Autodesk Fusion 360 part; units mm, degrees
(part 4 of 8)
  line L112 (-117.1979, 4.132) -> (-121.8798, -2.8001)
  spline S456 degree 3 poles (-131.6156, -11.2139) (-132.3559, -11.2139) (-133.0961, -11.2403) (-133.4953, -11.2934) knots 0 0 0 0 1 1 1 1
  spline S457 degree 3 poles (-133.4953, -11.2934) (-133.0961, -11.2403) (-132.3559, -11.2139) (-131.6156, -11.2139) knots -1 -1 -1 -1 0 0 0 0
  spline S458 degree 3 poles (188.5245, 6.5131) (188.7626, 6.5131) (189.0272, 5.9575) (189.0272, 5.64) knots 0 0 0 0 1 1 1 1
  spline S459 degree 3 poles (189.0272, 5.64) (189.0272, 5.9575) (188.7626, 6.5131) (188.5245, 6.5131) knots -1 -1 -1 -1 0 0 0 0
  spline S460 degree 3 poles (159.7907, 5.6135) (159.7907, 5.9575) (160.0818, 6.5131) (160.2934, 6.5131) knots 0 0 0 0 1 1 1 1
  spline S461 degree 3 poles (160.2934, 6.5131) (160.0818, 6.5131) (159.7907, 5.9575) (159.7907, 5.6135) knots -1 -1 -1 -1 0 0 0 0
  spline S462 degree 3 poles (213.7393, -9.3619) (215.3268, -9.3619) (215.6707, -9.4148) (215.6707, -8.7798) knots 0 0 0 0 1 1 1 1
  line L113 (215.6707, -8.7798) -> (215.6707, -3.1442)
  line L114 (215.6707, -3.1442) -> (213.8186, -3.1971)
  spline S463 degree 3 poles (213.8186, -3.1971) (211.6491, -3.25) (211.8078, -5.9753) (211.0141, -5.9753) knots 0 0 0 0 1 1 1 1
  spline S464 degree 3 poles (211.0141, -5.9753) (210.6966, -5.9753) (210.1145, -5.6842) (210.1145, -5.4725) knots 0 0 0 0 1 1 1 1
  spline S465 degree 3 poles (210.1145, -5.4725) (210.2468, -3.303) (210.2468, -1.1334) (210.1145, 1.0362) knots 0 0 0 0 1 1 1 1
  spline S466 degree 3 poles (210.1145, 1.0362) (210.1145, 1.2479) (210.6966, 1.5389) (211.0141, 1.5389) knots 0 0 0 0 1 1 1 1
  spline S467 degree 3 poles (211.0141, 1.5389) (211.8078, 1.5389) (211.6491, -1.1863) (213.8186, -1.2392) knots 0 0 0 0 1 1 1 1
  line L115 (213.8186, -1.2392) -> (215.6707, -1.2921)
  line L116 (215.6707, -1.2921) -> (215.6707, 4.1583)
  spline S468 degree 3 poles (215.6707, 4.1583) (215.6707, 5.296) (214.2155, 5.2166) (214.2155, 5.6135) knots 0 0 0 0 1 1 1 1
  spline S469 degree 3 poles (214.2155, 5.6135) (214.2155, 5.9575) (214.5066, 6.5131) (214.7182, 6.5131) knots 0 0 0 0 1 1 1 1
  spline S470 degree 3 poles (214.7182, 6.5131) (215.7501, 6.4602) (217.0466, 6.4337) (218.3166, 6.4337) knots 0 0 0 0 1 1 1 1
  spline S471 degree 3 poles (218.3166, 6.4337) (219.613, 6.4337) (220.883, 6.4602) (221.9414, 6.5131) knots 0 0 0 0 1 1 1 1
  spline S472 degree 3 poles (221.9414, 6.5131) (222.1795, 6.5131) (222.4441, 5.9575) (222.4441, 5.64) knots 0 0 0 0 1 1 1 1
  spline S473 degree 3 poles (222.4441, 5.64) (222.4441, 5.2166) (221.0153, 5.296) (221.0153, 4.1583) knots 0 0 0 0 1 1 1 1
  line L117 (221.0153, 4.1583) -> (221.0153, -8.9386)
  spline S474 degree 3 poles (221.0153, -8.9386) (221.0153, -10.0763) (222.4441, -9.9969) (222.4441, -10.3938) knots 0 0 0 0 1 1 1 1
  spline S475 degree 3 poles (222.4441, -10.3938) (222.4441, -10.7113) (222.1795, -11.2934) (221.9414, -11.2934) knots 0 0 0 0 1 1 1 1
  spline S476 degree 3 poles (221.9414, -11.2934) (220.1951, -11.2405) (217.7874, -11.214) (215.3532, -11.214) knots 0 0 0 0 1 1 1 1
  spline S477 degree 3 poles (215.3532, -11.214) (212.628, -11.214) (209.8764, -11.2405) (207.9184, -11.2934) knots 0 0 0 0 1 1 1 1
  spline S478 degree 3 poles (207.9184, -11.2934) (207.3893, -11.3225) (207.0718, -11.1611) (207.0718, -10.6848) knots 0 0 0 0 1 1 1 1
  spline S479 degree 3 poles (207.0718, -10.6848) (207.0718, -10.1028) (207.4951, -6.9807) (207.4951, -6.769) knots 0 0 0 0 1 1 1 1
  spline S480 degree 3 poles (207.4951, -6.769) (207.4951, -6.5573) (208.0507, -6.2663) (208.3682, -6.2663) knots 0 0 0 0 1 1 1 1
  spline S481 degree 3 poles (208.3682, -6.2663) (208.8709, -6.2663) (208.9503, -9.3619) (213.7393, -9.3619) knots 0 0 0 0 1 1 1 1
  spline S482 degree 3 poles (110.3163, 6.4337) (111.0571, 6.4337) (111.798, 6.4602) (112.1948, 6.5131) knots 0 0 0 0 1 1 1 1
  spline S483 degree 3 poles (112.1948, 6.5131) (111.798, 6.4602) (111.0571, 6.4337) (110.3163, 6.4337) knots -1 -1 -1 -1 0 0 0 0
  spline S484 degree 3 poles (106.0036, -11.2934) (105.104, -11.2934) (104.8394, -11.1346) (104.6542, -10.6584) knots 0 0 0 0 1 1 1 1
  spline S485 degree 3 poles (104.6542, -10.6584) (104.8394, -11.1346) (105.104, -11.2934) (106.0036, -11.2934) knots -1 -1 -1 -1 0 0 0 0
  spline S486 degree 3 poles (213.7393, -9.3619) (215.3268, -9.3619) (215.6707, -9.4148) (215.6707, -8.7798) knots 0 0 0 0 1 1 1 1
  spline S487 degree 3 poles (215.6707, -8.7798) (215.6707, -9.4148) (215.3268, -9.3619) (213.7393, -9.3619) knots -1 -1 -1 -1 0 0 0 0
  spline S488 degree 3 poles (177.3326, 5.64) (177.3326, 5.2166) (175.9039, 5.296) (175.9039, 4.1583) knots 0 0 0 0 1 1 1 1
  spline S489 degree 3 poles (175.9039, 4.1583) (175.9039, 5.296) (177.3326, 5.2166) (177.3326, 5.64) knots -1 -1 -1 -1 0 0 0 0
  spline S490 degree 3 poles (181.3014, -11.2934) (181.0897, -11.3225) (180.7986, -10.7378) (180.7986, -10.4203) knots 0 0 0 0 1 1 1 1
  spline S491 degree 3 poles (180.7986, -10.4203) (180.7986, -10.7378) (181.0897, -11.3225) (181.3014, -11.2934) knots -1 -1 -1 -1 0 0 0 0
  spline S492 degree 3 poles (-119.8955, 6.5132) (-119.4963, 6.4601) (-118.756, 6.4338) (-118.0157, 6.4338) knots 0 0 0 0 1 1 1 1
  spline S493 degree 3 poles (-118.0157, 6.4338) (-118.756, 6.4338) (-119.4963, 6.4601) (-119.8955, 6.5132) knots -1 -1 -1 -1 0 0 0 0
  line L118 (-132.8326, 4.1584) -> (-128.3096, -2.7738)
  line L119 (-128.3096, -2.7738) -> (-132.8326, 4.1584)
  spline S494 degree 3 poles (95.6584, -10.6584) (95.4732, -11.1346) (95.235, -11.2934) (94.309, -11.2934) knots 0 0 0 0 1 1 1 1
  spline S495 degree 3 poles (94.309, -11.2934) (95.235, -11.2934) (95.4732, -11.1346) (95.6584, -10.6584) knots -1 -1 -1 -1 0 0 0 0
  spline S496 degree 3 poles (163.9182, 6.4337) (165.2147, 6.4337) (166.4873, 6.4602) (167.5457, 6.5131) knots 0 0 0 0 1 1 1 1
  spline S497 degree 3 poles (167.5457, 6.5131) (166.4873, 6.4602) (165.2147, 6.4337) (163.9182, 6.4337) knots -1 -1 -1 -1 0 0 0 0
  spline S498 degree 3 poles (211.0141, -5.9753) (210.6966, -5.9753) (210.1145, -5.6842) (210.1145, -5.4725) knots 0 0 0 0 1 1 1 1
  spline S499 degree 3 poles (210.1145, -5.4725) (210.1145, -5.6842) (210.6966, -5.9753) (211.0141, -5.9753) knots -1 -1 -1 -1 0 0 0 0
  spline S500 degree 3 poles (102.0084, 6.4337) (102.6698, 6.4337) (103.3313, 6.4602) (104.2573, 6.5131) knots 0 0 0 0 1 1 1 1
  spline S501 degree 3 poles (104.2573, 6.5131) (103.3313, 6.4602) (102.6698, 6.4337) (102.0084, 6.4337) knots -1 -1 -1 -1 0 0 0 0
  spline S502 degree 3 poles (-4.0362, 6.4867) (-2.3431, 6.4867) (-3.3764, 5.8779) (-2.1844, 4.1319) knots 0 0 0 0 1 1 1 1
  spline S503 degree 3 poles (-2.1844, 4.1319) (-3.3764, 5.8779) (-2.3431, 6.4867) (-4.0362, 6.4867) knots -1 -1 -1 -1 0 0 0 0
  spline S504 degree 3 poles (221.9414, -11.2934) (220.1951, -11.2405) (217.7874, -11.214) (215.3532, -11.214) knots 0 0 0 0 1 1 1 1
  spline S505 degree 3 poles (215.3532, -11.214) (217.7874, -11.214) (220.1951, -11.2405) (221.9414, -11.2934) knots -1 -1 -1 -1 0 0 0 0
  spline S506 degree 3 poles (168.0193, 5.64) (168.0193, 5.2166) (166.5905, 5.296) (166.5905, 4.1583) knots 0 0 0 0 1 1 1 1
  spline S507 degree 3 poles (166.5905, 4.1583) (166.5905, 5.296) (168.0193, 5.2166) (168.0193, 5.64) knots -1 -1 -1 -1 0 0 0 0
  spline S508 degree 3 poles (94.309, -11.2934) (93.4094, -11.2934) (91.6367, -11.1346) (89.7317, -11.2934) knots 0 0 0 0 1 1 1 1
  spline S509 degree 3 poles (89.7317, -11.2934) (91.6367, -11.1346) (93.4094, -11.2934) (94.309, -11.2934) knots -1 -1 -1 -1 0 0 0 0
  spline S510 degree 3 poles (160.2934, 6.5131) (161.3253, 6.4602) (162.6218, 6.4337) (163.9182, 6.4337) knots 0 0 0 0 1 1 1 1
  spline S511 degree 3 poles (163.9182, 6.4337) (162.6218, 6.4337) (161.3253, 6.4602) (160.2934, 6.5131) knots -1 -1 -1 -1 0 0 0 0
  spline S512 degree 3 poles (167.5457, -11.2934) (166.4873, -11.2405) (165.2147, -11.214) (163.9182, -11.214) knots 0 0 0 0 1 1 1 1
  spline S513 degree 3 poles (163.9182, -11.214) (165.2147, -11.214) (166.4873, -11.2405) (167.5457, -11.2934) knots -1 -1 -1 -1 0 0 0 0
  spline S514 degree 3 poles (-63.4057, -10.3935) (-63.4057, -10.5655) (-63.4913, -10.8075) (-63.6031, -10.9931) knots 0 0 0 0 0.541892 0.541892 0.541892 0.541892
  spline S515 degree 3 poles (-63.6031, -10.9931) (-63.4913, -10.8075) (-63.4057, -10.5655) (-63.4057, -10.3935) knots -0.541892 -0.541892 -0.541892 -0.541892 0 0 0 0
  spline S516 degree 3 poles (-79.7806, -11.1902) (-80.577, -11.1902) (-81.3698, -11.2136) (-81.768, -11.2666) knots 0 0 0 0 1 1 1 1
  spline S517 degree 3 poles (-81.768, -11.2666) (-81.3698, -11.2136) (-80.577, -11.1902) (-79.7806, -11.1902) knots -1 -1 -1 -1 0 0 0 0
  spline S518 degree 5 poles (-63.6031, -10.9931) (-63.6143, -11.005) (-63.6642, -11.057) (-63.7203, -11.1105) (-63.7825, -11.1656) (-63.8508, -11.2222) (-63.907, -11.2666) knots 0.913312 0.913312 0.913312 0.913312 0.913312 0.913312 0.933333 1 1 1 1 1 1
  spline S519 degree 5 poles (-63.907, -11.2666) (-63.8508, -11.2222) (-63.7825, -11.1656) (-63.7203, -11.1105) (-63.6642, -11.057) (-63.6143, -11.005) (-63.6031, -10.9931) knots -1 -1 -1 -1 -1 -1 -0.933333 -0.913312 -0.913312 -0.913312 -0.913312 -0.913312 -0.913312
  spline S520 degree 3 poles (-44.0427, -6.2399) (-44.0427, -6.0282) (-43.4578, -5.7371) (-43.1421, -5.7371) knots 0 0 0 0 1 1 1 1
  spline S521 degree 3 poles (-43.1421, -5.7371) (-43.4578, -5.7371) (-44.0427, -6.0282) (-44.0427, -6.2399) knots -1 -1 -1 -1 0 0 0 0
  spline S522 degree 3 poles (23.2168, -2.3771) (23.2168, -7.2718) (22.1298, -9.7058) (19.7498, -9.7058) knots -1 -1 -1 -1 0 0 0 0
  spline S523 degree 3 poles (23.2168, -2.3771) (23.2168, -7.2718) (22.1298, -9.7058) (19.7498, -9.7058) knots -1 -1 -1 -1 0 0 0 0
  line L120 (-37.7953, 4.1582) -> (-37.7953, -8.7797)
  line L121 (-37.7953, -8.7797) -> (-37.7953, 4.1582)
  spline S524 degree 3 poles (19.7498, 4.9254) (22.1298, 4.9254) (23.2168, 2.518) (23.2168, -2.3771) knots -1 -1 -1 -1 0 0 0 0
  spline S525 degree 3 poles (19.7498, 4.9254) (22.1298, 4.9254) (23.2168, 2.518) (23.2168, -2.3771) knots -1 -1 -1 -1 0 0 0 0
  spline S526 degree 3 poles (-38.6427, -9.3619) (-38.111, -9.3619) (-37.7953, -9.4413) (-37.7953, -8.7797) knots 0 0 0 0 1 1 1 1
  line L122 (-37.7953, -8.7797) -> (-37.7953, 4.1582)
  spline S527 degree 3 poles (-37.7953, 4.1582) (-37.7953, 5.296) (-39.2508, 5.2166) (-39.2508, 5.6137) knots 0 0 0 0 1 1 1 1
  spline S528 degree 3 poles (-39.2508, 5.6137) (-39.2508, 5.931) (-38.9584, 6.5132) (-38.7457, 6.5132) knots 0 0 0 0 1 1 1 1
  spline S529 degree 3 poles (-38.7457, 6.5132) (-37.7156, 6.46) (-36.4196, 6.4338) (-35.1236, 6.4338) knots 0 0 0 0 1 1 1 1
  spline S530 degree 3 poles (-35.1236, 6.4338) (-33.8243, 6.4338) (-32.5549, 6.46) (-31.4982, 6.5132) knots 0 0 0 0 1 1 1 1
  spline S531 degree 3 poles (-31.4982, 6.5132) (-31.2855, 6.5132) (-31.0197, 5.931) (-31.0197, 5.6137) knots 0 0 0 0 1 1 1 1
  spline S532 degree 3 poles (-31.0197, 5.6137) (-31.0197, 5.2166) (-32.4486, 5.296) (-32.4486, 4.1582) knots 0 0 0 0 1 1 1 1
  line L123 (-32.4486, 4.1582) -> (-32.4486, -8.7797)
  spline S533 degree 3 poles (-32.4486, -8.7797) (-32.4486, -9.1768) (-32.1329, -9.3619) (-31.4184, -9.3619) knots 0 0 0 0 1 1 1 1
  spline S534 degree 3 poles (-31.4184, -9.3619) (-28.3745, -9.3619) (-27.1051, -5.7372) (-26.6033, -5.7372) knots 0 0 0 0 1 1 1 1
  spline S535 degree 3 poles (-26.6033, -5.7372) (-26.2843, -5.7372) (-25.7028, -6.0017) (-25.7028, -6.2399) knots 0 0 0 0 1 1 1 1
  spline S536 degree 3 poles (-25.7028, -6.2399) (-25.7028, -6.4516) (-26.2046, -10.1292) (-26.2578, -10.4731) knots 0 0 0 0 1 1 1 1
  spline S537 degree 3 poles (-26.2578, -10.4731) (-26.3641, -11.161) (-26.63, -11.3225) (-27.1849, -11.2933) knots 0 0 0 0 1 1 1 1
  spline S538 degree 3 poles (-27.1849, -11.2933) (-29.9364, -11.2404) (-32.6613, -11.2138) (-35.3861, -11.2138) knots 0 0 0 0 1 1 1 1
  spline S539 degree 3 poles (-35.3861, -11.2138) (-38.111, -11.2138) (-40.8658, -11.2404) (-43.5907, -11.2933) knots 0 0 0 0 1 1 1 1
  spline S540 degree 3 poles (-43.5907, -11.2933) (-44.1191, -11.3225) (-44.4381, -11.161) (-44.4381, -10.6848) knots 0 0 0 0 1 1 1 1
  spline S541 degree 3 poles (-44.4381, -10.6848) (-44.4381, -10.1292) (-44.0427, -6.4516) (-44.0427, -6.2399) knots 0 0 0 0 1 1 1 1
  spline S542 degree 3 poles (-44.0427, -6.2399) (-44.0427, -6.0282) (-43.4578, -5.7371) (-43.1421, -5.7371) knots 0 0 0 0 1 1 1 1
  spline S543 degree 3 poles (-43.1421, -5.7371) (-42.6404, -5.7371) (-42.4277, -9.3619) (-38.6427, -9.3619) knots 0 0 0 0 1 1 1 1
  spline S544 degree 3 poles (177.3326, -10.4203) (177.3326, -10.7378) (177.068, -11.3225) (176.8564, -11.2934) knots 0 0 0 0 1 1 1 1
  spline S545 degree 3 poles (176.8564, -11.2934) (177.068, -11.3225) (177.3326, -10.7378) (177.3326, -10.4203) knots -1 -1 -1 -1 0 0 0 0
  spline S546 degree 3 poles (11.3616, 8.4444) (11.3616, 10.4553) (12.9234, 12.1751) (15.2526, 12.1222) knots 0 0 0 0 1 1 1 1
  spline S547 degree 3 poles (15.2526, 12.1222) (12.9234, 12.1751) (11.3616, 10.4553) (11.3616, 8.4444) knots -1 -1 -1 -1 0 0 0 0
  spline S548 degree 3 poles (-25.7028, -6.2399) (-25.7028, -6.4516) (-26.2046, -10.1292) (-26.2578, -10.4731) knots 0 0 0 0 1 1 1 1
  spline S549 degree 3 poles (-26.2578, -10.4731) (-26.2046, -10.1292) (-25.7028, -6.4516) (-25.7028, -6.2399) knots -1 -1 -1 -1 0 0 0 0
  spline S550 degree 3 poles (24.1426, 7.307) (24.8832, 7.307) (25.2803, 7.8624) (25.2803, 8.4181) knots 0 0 0 0 1 1 1 1
  spline S551 degree 3 poles (25.2803, 8.4181) (25.2803, 7.8624) (24.8832, 7.307) (24.1426, 7.307) knots -1 -1 -1 -1 0 0 0 0
  spline S552 degree 3 poles (19.5885, -11.5568) (19.4017, -11.5543) (19.2169, -11.5473) (19.0342, -11.5361) knots 0.009853 0.009853 0.009853 0.009853 0.044162 0.044162 0.044162 0.044162
  spline S553 degree 3 poles (19.0342, -11.5361) (19.2169, -11.5473) (19.4017, -11.5543) (19.5885, -11.5568) knots -0.044162 -0.044162 -0.044162 -0.044162 -0.009853 -0.009853 -0.009853 -0.009853
  spline S554 degree 3 poles (-31.0197, 5.6137) (-31.0197, 5.2166) (-32.4486, 5.296) (-32.4486, 4.1582) knots 0 0 0 0 1 1 1 1
  spline S555 degree 3 poles (-32.4486, 4.1582) (-32.4486, 5.296) (-31.0197, 5.2166) (-31.0197, 5.6137) knots -1 -1 -1 -1 0 0 0 0
  spline S556 degree 3 poles (215.6707, 4.1583) (215.6707, 5.296) (214.2155, 5.2166) (214.2155, 5.6135) knots 0 0 0 0 1 1 1 1
  spline S557 degree 3 poles (214.2155, 5.6135) (214.2155, 5.2166) (215.6707, 5.296) (215.6707, 4.1583) knots -1 -1 -1 -1 0 0 0 0
  spline S558 degree 3 poles (-21.7884, -11.0288) (-22.4483, -11.0288) (-22.6342, -11.2934) (-23.0859, -11.2934) knots 0 0 0 0 1 1 1 1
  spline S559 degree 3 poles (-23.0859, -11.2934) (-22.6342, -11.2934) (-22.4483, -11.0288) (-21.7884, -11.0288) knots -1 -1 -1 -1 0 0 0 0
  spline S560 degree 3 poles (299.0115, 4.1318) (298.6411, 5.2166) (297.4505, 5.1902) (297.4505, 5.587) knots 0 0 0 0 1 1 1 1
  spline S561 degree 3 poles (297.4505, 5.587) (297.4505, 5.1902) (298.6411, 5.2166) (299.0115, 4.1318) knots -1 -1 -1 -1 0 0 0 0
  line L124 (-128.3096, -2.7738) -> (-132.4373, -8.9121)
  line L125 (-132.4373, -8.9121) -> (-128.3096, -2.7738)
  line L126 (-52.1084, -0.3134) -> (-52.1084, -8.9652)
  line L127 (-52.1084, -8.9652) -> (-52.1084, -0.3134)
  spline S562 degree 3 poles (-53.0631, -11.2935) (-53.2726, -11.2935) (-53.5645, -10.7379) (-53.5645, -10.4202) knots 0 0 0 0 1 1 1 1
  spline S563 degree 3 poles (-53.5645, -10.4202) (-53.5645, -10.7379) (-53.2726, -11.2935) (-53.0631, -11.2935) knots -1 -1 -1 -1 0 0 0 0
  line L128 (161.2459, 4.1583) -> (161.2459, -8.965)
  line L129 (161.2459, -8.965) -> (161.2459, 4.1583)
  line L130 (-78.5932, -8.9383) -> (-74.6506, 2.4388)
  line L131 (-74.6506, 2.4388) -> (-78.5932, -8.9383)
  line L132 (8.0583, -8.9652) -> (8.0583, 4.1848)
  line L133 (8.0583, 4.1848) -> (8.0583, -8.9652)
  spline S564 degree 3 poles (184.8997, -11.214) (183.6297, -11.214) (182.3332, -11.2405) (181.3014, -11.2934) knots 0 0 0 0 1 1 1 1
  spline S565 degree 3 poles (181.3014, -11.2934) (182.3332, -11.2405) (183.6297, -11.214) (184.8997, -11.214) knots -1 -1 -1 -1 0 0 0 0
  line L134 (187.5984, -8.965) -> (187.5984, 4.1583)
  line L135 (187.5984, 4.1583) -> (187.5984, -8.965)
  spline S566 degree 3 poles (221.9414, 6.5131) (222.1795, 6.5131) (222.4441, 5.9575) (222.4441, 5.64) knots 0 0 0 0 1 1 1 1
  spline S567 degree 3 poles (222.4441, 5.64) (222.4441, 5.9575) (222.1795, 6.5131) (221.9414, 6.5131) knots -1 -1 -1 -1 0 0 0 0
  spline S568 degree 3 poles (182.2539, 4.1583) (182.2539, 5.296) (180.7986, 5.2166) (180.7986, 5.64) knots 0 0 0 0 1 1 1 1
  spline S569 degree 3 poles (180.7986, 5.64) (180.7986, 5.2166) (182.2539, 5.296) (182.2539, 4.1583) knots -1 -1 -1 -1 0 0 0 0
  line L136 (109.3902, 4.1583) -> (108.2261, -4.7317)
  line L137 (108.2261, -4.7317) -> (109.3902, 4.1583)
  line L138 (213.8186, -3.1971) -> (215.6707, -3.1442)
  line L139 (215.6707, -3.1442) -> (213.8186, -3.1971)
  line L140 (0.9622, -0.5248) -> (-2.1844, 4.1319)
  line L141 (-2.1844, 4.1319) -> (0.9622, -0.5248)
  spline S570 degree 3 poles (207.9184, -11.2934) (207.3893, -11.3225) (207.0718, -11.1611) (207.0718, -10.6848) knots 0 0 0 0 1 1 1 1
  spline S571 degree 3 poles (207.0718, -10.6848) (207.0718, -11.1611) (207.3893, -11.3225) (207.9184, -11.2934) knots -1 -1 -1 -1 0 0 0 0
  line L142 (95.6584, -10.6584) -> (100.1563, 1.6977)
  line L143 (100.1563, 1.6977) -> (95.6584, -10.6584)
  line L144 (166.5905, -8.965) -> (166.5905, 4.1583)
  line L145 (166.5905, 4.1583) -> (166.5905, -8.965)
  spline S572 degree 3 poles (213.8186, -3.1971) (211.6491, -3.25) (211.8078, -5.9753) (211.0141, -5.9753) knots 0 0 0 0 1 1 1 1
  spline S573 degree 3 poles (211.0141, -5.9753) (211.8078, -5.9753) (211.6491, -3.25) (213.8186, -3.1971) knots -1 -1 -1 -1 0 0 0 0
  spline S574 degree 3 poles (9.0107, 6.5131) (9.2223, 6.5131) (9.5118, 5.9573) (9.5118, 5.6398) knots 0 0 0 0 1 1 1 1
  spline S575 degree 3 poles (9.5118, 5.6398) (9.5118, 5.9573) (9.2223, 6.5131) (9.0107, 6.5131) knots -1 -1 -1 -1 0 0 0 0
  spline S576 degree 3 poles (-129.7359, -11.2934) (-130.1351, -11.2403) (-130.8754, -11.2139) (-131.6156, -11.2139) knots 0 0 0 0 1 1 1 1
  spline S577 degree 3 poles (-131.6156, -11.2139) (-130.8754, -11.2139) (-130.1351, -11.2403) (-129.7359, -11.2934) knots -1 -1 -1 -1 0 0 0 0
  spline S578 degree 3 poles (173.2316, 6.4337) (174.5016, 6.4337) (175.798, 6.4602) (176.8564, 6.5131) knots 0 0 0 0 1 1 1 1
  spline S579 degree 3 poles (176.8564, 6.5131) (175.798, 6.4602) (174.5016, 6.4337) (173.2316, 6.4337) knots -1 -1 -1 -1 0 0 0 0
  spline S580 degree 3 poles (-37.7953, -8.7797) (-37.7953, -9.4413) (-38.111, -9.3619) (-38.6427, -9.3619) knots -1 -1 -1 -1 0 0 0 0
  spline S581 degree 3 poles (-38.6427, -9.3619) (-42.4277, -9.3619) (-42.6404, -5.7371) (-43.1421, -5.7371) knots -1 -1 -1 -1 0 0 0 0
  spline S582 degree 3 poles (-43.1421, -5.7371) (-43.4578, -5.7371) (-44.0427, -6.0282) (-44.0427, -6.2399) knots -1 -1 -1 -1 0 0 0 0
  spline S583 degree 3 poles (-44.0427, -6.2399) (-44.0427, -6.4516) (-44.4381, -10.1292) (-44.4381, -10.6848) knots -1 -1 -1 -1 0 0 0 0
  spline S584 degree 3 poles (-44.4381, -10.6848) (-44.4381, -11.161) (-44.1191, -11.3225) (-43.5907, -11.2933) knots -1 -1 -1 -1 0 0 0 0
  spline S585 degree 3 poles (-43.5907, -11.2933) (-40.8658, -11.2404) (-38.111, -11.2138) (-35.3861, -11.2138) knots -1 -1 -1 -1 0 0 0 0
  spline S586 degree 3 poles (-35.3861, -11.2138) (-32.6613, -11.2138) (-29.9364, -11.2404) (-27.1849, -11.2933) knots -1 -1 -1 -1 0 0 0 0
  spline S587 degree 3 poles (-27.1849, -11.2933) (-26.63, -11.3225) (-26.3641, -11.161) (-26.2578, -10.4731) knots -1 -1 -1 -1 0 0 0 0
  spline S588 degree 3 poles (-26.2578, -10.4731) (-26.2046, -10.1292) (-25.7028, -6.4516) (-25.7028, -6.2399) knots -1 -1 -1 -1 0 0 0 0
  spline S589 degree 3 poles (-25.7028, -6.2399) (-25.7028, -6.0017) (-26.2843, -5.7372) (-26.6033, -5.7372) knots -1 -1 -1 -1 0 0 0 0
  spline S590 degree 3 poles (-26.6033, -5.7372) (-27.1051, -5.7372) (-28.3745, -9.3619) (-31.4184, -9.3619) knots -1 -1 -1 -1 0 0 0 0
  spline S591 degree 3 poles (-31.4184, -9.3619) (-32.1329, -9.3619) (-32.4486, -9.1768) (-32.4486, -8.7797) knots -1 -1 -1 -1 0 0 0 0
  line L146 (-32.4486, -8.7797) -> (-32.4486, 4.1582)
  spline S592 degree 3 poles (-32.4486, 4.1582) (-32.4486, 5.296) (-31.0197, 5.2166) (-31.0197, 5.6137) knots -1 -1 -1 -1 0 0 0 0
  spline S593 degree 3 poles (-31.0197, 5.6137) (-31.0197, 5.931) (-31.2855, 6.5132) (-31.4982, 6.5132) knots -1 -1 -1 -1 0 0 0 0
  spline S594 degree 3 poles (-31.4982, 6.5132) (-32.5549, 6.46) (-33.8243, 6.4338) (-35.1236, 6.4338) knots -1 -1 -1 -1 0 0 0 0
  spline S595 degree 3 poles (-35.1236, 6.4338) (-36.4196, 6.4338) (-37.7156, 6.46) (-38.7457, 6.5132) knots -1 -1 -1 -1 0 0 0 0
  spline S596 degree 3 poles (-38.7457, 6.5132) (-38.9584, 6.5132) (-39.2508, 5.931) (-39.2508, 5.6137) knots -1 -1 -1 -1 0 0 0 0
  spline S597 degree 3 poles (-39.2508, 5.6137) (-39.2508, 5.2166) (-37.7953, 5.296) (-37.7953, 4.1582) knots -1 -1 -1 -1 0 0 0 0
  line L147 (-37.7953, 4.1582) -> (-37.7953, -8.7797)
  spline S598 degree 3 poles (12.3354, 3.4367) (13.6571, 5.1309) (15.615, 6.2706) (18.0029, 6.6455) knots 0.475314 0.475314 0.475314 0.475314 1 1 1 1
  spline S599 degree 3 poles (18.0029, 6.6455) (15.615, 6.2706) (13.6571, 5.1309) (12.3354, 3.4367) knots -1 -1 -1 -1 -0.475314 -0.475314 -0.475314 -0.475314
  spline S600 degree 3 poles (24.3785, 5.7192) (25.0522, 5.3732) (25.6655, 4.9493) (26.2098, 4.4555) knots 0 0 0 0 0.233548 0.233548 0.233548 0.233548
  spline S601 degree 3 poles (26.2098, 4.4555) (25.6655, 4.9493) (25.0522, 5.3732) (24.3785, 5.7192) knots -0.233548 -0.233548 -0.233548 -0.233548 0 0 0 0
  spline S602 degree 3 poles (-38.6427, -9.3619) (-38.111, -9.3619) (-37.7953, -9.4413) (-37.7953, -8.7797) knots 0 0 0 0 1 1 1 1
  spline S603 degree 3 poles (-37.7953, -8.7797) (-37.7953, -9.4413) (-38.111, -9.3619) (-38.6427, -9.3619) knots -1 -1 -1 -1 0 0 0 0
  line L148 (-64.9913, -8.9383) -> (-70.4164, 6.5133)
  line L149 (-70.4164, 6.5133) -> (-64.9913, -8.9383)
  spline S604 degree 3 poles (-52.1084, -0.3134) (-52.1084, 2.7559) (-53.434, 4.3435) (-55.6798, 4.3435) knots 0 0 0 0 1 1 1 1
  spline S605 degree 3 poles (-55.6798, 4.3435) (-53.434, 4.3435) (-52.1084, 2.7559) (-52.1084, -0.3134) knots -1 -1 -1 -1 0 0 0 0
  spline S606 degree 3 poles (176.8564, 6.5131) (177.068, 6.5131) (177.3326, 5.9575) (177.3326, 5.64) knots 0 0 0 0 1 1 1 1
  spline S607 degree 3 poles (177.3326, 5.64) (177.3326, 5.9575) (177.068, 6.5131) (176.8564, 6.5131) knots -1 -1 -1 -1 0 0 0 0
  spline S608 degree 3 poles (-32.4486, -8.7797) (-32.4486, -9.1768) (-32.1329, -9.3619) (-31.4184, -9.3619) knots 0 0 0 0 1 1 1 1
  spline S609 degree 3 poles (-31.4184, -9.3619) (-32.1329, -9.3619) (-32.4486, -9.1768) (-32.4486, -8.7797) knots -1 -1 -1 -1 0 0 0 0
  spline S610 degree 3 poles (170.5593, 4.1583) (170.5593, 5.296) (169.1041, 5.2166) (169.1041, 5.64) knots 0 0 0 0 1 1 1 1
  spline S611 degree 3 poles (169.1041, 5.64) (169.1041, 5.2166) (170.5593, 5.296) (170.5593, 4.1583) knots -1 -1 -1 -1 0 0 0 0
  spline S612 degree 3 poles (-133.9953, -10.4202) (-133.9953, -9.9969) (-133.0729, -9.8648) (-132.4373, -8.9121) knots 0 0 0 0 1 1 1 1
  spline S613 degree 3 poles (-132.4373, -8.9121) (-133.0729, -9.8648) (-133.9953, -9.9969) (-133.9953, -10.4202) knots -1 -1 -1 -1 0 0 0 0
  line L150 (182.2539, 4.1583) -> (182.2539, -1.9007)
  line L151 (182.2539, -1.9007) -> (182.2539, 4.1583)
  spline S614 degree 3 poles (169.1041, 5.64) (169.1041, 5.9575) (169.3951, 6.5131) (169.6068, 6.5131) knots 0 0 0 0 1 1 1 1
  spline S615 degree 3 poles (169.6068, 6.5131) (169.3951, 6.5131) (169.1041, 5.9575) (169.1041, 5.64) knots -1 -1 -1 -1 0 0 0 0
  line L152 (182.2539, -1.9007) -> (175.9039, -1.9007)
  line L153 (175.9039, -1.9007) -> (182.2539, -1.9007)
  spline S616 degree 3 poles (169.6068, 6.5131) (170.6386, 6.4602) (171.9351, 6.4337) (173.2316, 6.4337) knots 0 0 0 0 1 1 1 1
  spline S617 degree 3 poles (173.2316, 6.4337) (171.9351, 6.4337) (170.6386, 6.4602) (169.6068, 6.5131) knots -1 -1 -1 -1 0 0 0 0
  line L154 (175.9039, -1.9007) -> (175.9039, 4.1583)
  line L155 (175.9039, 4.1583) -> (175.9039, -1.9007)
  spline S618 degree 3 poles (-118.0157, 6.4338) (-117.2755, 6.4338) (-116.5352, 6.4601) (-116.136, 6.5132) knots 0 0 0 0 1 1 1 1
  spline S619 degree 3 poles (-116.136, 6.5132) (-116.5352, 6.4601) (-117.2755, 6.4338) (-118.0157, 6.4338) knots -1 -1 -1 -1 0 0 0 0
  spline S620 degree 3 poles (161.2459, 4.1583) (161.2459, 5.296) (159.7907, 5.2166) (159.7907, 5.6135) knots 0 0 0 0 1 1 1 1
  spline S621 degree 3 poles (159.7907, 5.6135) (159.7907, 5.2166) (161.2459, 5.296) (161.2459, 4.1583) knots -1 -1 -1 -1 0 0 0 0
  line L156 (109.7077, -8.9386) -> (111.3746, 4.1583)
  spline S622 degree 3 poles (111.3746, 4.1583) (111.5334, 5.296) (112.6975, 5.2166) (112.6975, 5.6135) knots -1 -1 -1 -1 0 0 0 0
  spline S623 degree 3 poles (112.6975, 5.6135) (112.6975, 5.931) (112.4065, 6.5395) (112.1948, 6.5131) knots -1 -1 -1 -1 0 0 0 0
  spline S624 degree 3 poles (112.1948, 6.5131) (111.798, 6.4602) (111.0571, 6.4337) (110.3163, 6.4337) knots -1 -1 -1 -1 0 0 0 0
  spline S625 degree 3 poles (110.3163, 6.4337) (109.5755, 6.4337) (108.8346, 6.4602) (108.4377, 6.5131) knots -1 -1 -1 -1 0 0 0 0
  spline S626 degree 3 poles (108.4377, 6.5131) (108.2261, 6.5395) (107.9615, 5.931) (107.9615, 5.6135) knots -1 -1 -1 -1 0 0 0 0
  spline S627 degree 3 poles (107.9615, 5.6135) (107.9615, 5.2166) (109.549, 5.296) (109.3902, 4.1583) knots -1 -1 -1 -1 0 0 0 0
  line L157 (109.3902, 4.1583) -> (108.2261, -4.7317)
  line L158 (108.2261, -4.7317) -> (104.2573, 6.5131)
  spline S628 degree 3 poles (104.2573, 6.5131) (103.3313, 6.4602) (102.6698, 6.4337) (102.0084, 6.4337) knots -1 -1 -1 -1 0 0 0 0
  spline S629 degree 3 poles (102.0084, 6.4337) (101.3469, 6.4337) (100.6855, 6.4602) (99.7859, 6.5131) knots -1 -1 -1 -1 0 0 0 0
  line L159 (99.7859, 6.5131) -> (95.7113, -4.7053)
  line L160 (95.7113, -4.7053) -> (94.7323, 4.1583)
  spline S630 degree 3 poles (94.7323, 4.1583) (94.6265, 5.296) (96.1875, 5.2166) (96.1875, 5.6135) knots -1 -1 -1 -1 0 0 0 0
  spline S631 degree 3 poles (96.1875, 5.6135) (96.1875, 5.931) (95.8965, 6.5395) (95.6848, 6.5131) knots -1 -1 -1 -1 0 0 0 0
  spline S632 degree 3 poles (95.6848, 6.5131) (95.288, 6.4602) (93.7005, 6.4337) (92.1394, 6.4337) knots -1 -1 -1 -1 0 0 0 0
  spline S633 degree 3 poles (92.1394, 6.4337) (90.5519, 6.4337) (88.9644, 6.4602) (88.5675, 6.5131) knots -1 -1 -1 -1 0 0 0 0
  spline S634 degree 3 poles (88.5675, 6.5131) (88.3559, 6.5395) (88.0913, 5.931) (88.0913, 5.6135) knots -1 -1 -1 -1 0 0 0 0
  spline S635 degree 3 poles (88.0913, 5.6135) (88.0913, 5.2166) (89.2819, 5.296) (89.3877, 4.1583) knots -1 -1 -1 -1 0 0 0 0
  line L161 (89.3877, 4.1583) -> (90.8165, -8.9121)
  spline S636 degree 3 poles (90.8165, -8.9121) (90.9223, -10.0234) (89.2555, -9.9969) (89.2555, -10.4203) knots -1 -1 -1 -1 0 0 0 0
  spline S637 degree 3 poles (89.2555, -10.4203) (89.2555, -10.7378) (89.52, -11.3225) (89.7317, -11.2934) knots -1 -1 -1 -1 0 0 0 0
  spline S638 degree 3 poles (89.7317, -11.2934) (91.6367, -11.1346) (93.4094, -11.2934) (94.309, -11.2934) knots -1 -1 -1 -1 0 0 0 0
  spline S639 degree 3 poles (94.309, -11.2934) (95.235, -11.2934) (95.4732, -11.1346) (95.6584, -10.6584) knots -1 -1 -1 -1 0 0 0 0
  line L162 (95.6584, -10.6584) -> (100.1563, 1.6977)
  line L163 (100.1563, 1.6977) -> (104.6542, -10.6584)
  spline S640 degree 3 poles (104.6542, -10.6584) (104.8394, -11.1346) (105.104, -11.2934) (106.0036, -11.2934) knots -1 -1 -1 -1 0 0 0 0
  spline S641 degree 3 poles (106.0036, -11.2934) (106.9032, -11.2934) (108.914, -11.1346) (110.7925, -11.2934) knots -1 -1 -1 -1 0 0 0 0
  spline S642 degree 3 poles (110.7925, -11.2934) (111.0042, -11.3225) (111.2952, -10.7378) (111.2952, -10.4203) knots -1 -1 -1 -1 0 0 0 0
  spline S643 degree 3 poles (111.2952, -10.4203) (111.2952, -9.9969) (109.5755, -10.0498) (109.7077, -8.9386) knots -1 -1 -1 -1 0 0 0 0
  spline S644 degree 3 poles (-133.4953, -11.2934) (-133.7046, -11.3224) (-133.9953, -10.7376) (-133.9953, -10.4202) knots 0 0 0 0 1 1 1 1
  spline S645 degree 3 poles (-133.9953, -10.4202) (-133.9953, -10.7376) (-133.7046, -11.3224) (-133.4953, -11.2934) knots -1 -1 -1 -1 0 0 0 0
  spline S646 degree 3 poles (169.1041, -10.4203) (169.1041, -9.9969) (170.5593, -10.0763) (170.5593, -8.965) knots 0 0 0 0 1 1 1 1
  spline S647 degree 3 poles (170.5593, -8.965) (170.5593, -10.0763) (169.1041, -9.9969) (169.1041, -10.4203) knots -1 -1 -1 -1 0 0 0 0
  line L164 (312.7442, 4.1318) -> (311.8446, 1.6183)
  line L165 (311.8446, 1.6183) -> (312.7442, 4.1318)
  spline S648 degree 3 poles (305.5206, 6.4866) (305.7322, 6.4866) (306.0235, 5.9045) (306.0235, 5.587) knots 0 0 0 0 1 1 1 1
  spline S649 degree 3 poles (306.0235, 5.587) (306.0235, 5.9045) (305.7322, 6.4866) (305.5206, 6.4866) knots -1 -1 -1 -1 0 0 0 0
  spline S650 degree 3 poles (175.9039, -8.965) (175.9039, -10.0763) (177.3326, -9.9969) (177.3326, -10.4203) knots 0 0 0 0 1 1 1 1
  spline S651 degree 3 poles (177.3326, -10.4203) (177.3326, -9.9969) (175.9039, -10.0763) (175.9039, -8.965) knots -1 -1 -1 -1 0 0 0 0
  spline S652 degree 3 poles (-116.1631, -10.4202) (-116.1631, -10.7376) (-116.4538, -11.3224) (-116.6669, -11.2934) knots 0 0 0 0 1 1 1 1
  spline S653 degree 3 poles (-116.6669, -11.2934) (-116.4538, -11.3224) (-116.1631, -10.7376) (-116.1631, -10.4202) knots -1 -1 -1 -1 0 0 0 0
  spline S654 degree 3 poles (-130.0537, -8.9121) (-130.6622, -9.8648) (-129.1545, -9.9969) (-129.1545, -10.4202) knots 0 0 0 0 1 1 1 1
  spline S655 degree 3 poles (-129.1545, -10.4202) (-129.1545, -9.9969) (-130.6622, -9.8648) (-130.0537, -8.9121) knots -1 -1 -1 -1 0 0 0 0
  spline S656 degree 3 poles (-17.7132, 4.8726) (-19.2478, 4.8726) (-20.2282, 4.1848) (-20.2282, 3.0734) knots 0 0 0 0 1 1 1 1
  spline S657 degree 3 poles (-20.2282, 3.0734) (-20.1993, 0.0308) (-10.7804, 0.4806) (-10.7804, -6.1341) knots 0 0 0 0 1 1 1 1
  spline S658 degree 3 poles (-10.7804, -6.1341) (-10.7804, -9.4414) (-13.401, -11.5581) (-17.5018, -11.5581) knots 0 0 0 0 1 1 1 1
  spline S659 degree 3 poles (-17.5018, -11.5581) (-19.8821, -11.5581) (-20.8625, -11.0288) (-21.7884, -11.0288) knots 0 0 0 0 1 1 1 1
  spline S660 degree 3 poles (-21.7884, -11.0288) (-22.4483, -11.0288) (-22.6342, -11.2934) (-23.0859, -11.2934) knots 0 0 0 0 1 1 1 1
  spline S661 degree 3 poles (-23.0859, -11.2934) (-23.4287, -11.2934) (-23.6177, -10.976) (-23.7491, -10.4733) knots 0 0 0 0 1 1 1 1
  spline S662 degree 3 poles (-23.7491, -10.4733) (-23.8804, -10.0763) (-24.4347, -6.7163) (-24.4347, -6.5045) knots 0 0 0 0 1 1 1 1
  spline S663 degree 3 poles (-24.4347, -6.5045) (-24.4347, -6.2927) (-23.8804, -5.7372) (-23.5601, -5.7372) knots 0 0 0 0 1 1 1 1
  spline S664 degree 3 poles (-23.5601, -5.7372) (-23.0571, -5.7372) (-20.9682, -9.6531) (-17.8446, -9.6531) knots 0 0 0 0 1 1 1 1
  spline S665 degree 3 poles (-17.8446, -9.6531) (-16.5759, -9.6531) (-15.6244, -8.8858) (-15.6244, -7.8539) knots 0 0 0 0 1 1 1 1
  spline S666 degree 3 poles (-15.6244, -7.8539) (-15.6244, -4.5467) (-24.9921, -5.1022) (-24.9921, 1.3536) knots 0 0 0 0 1 1 1 1
  spline S667 degree 3 poles (-24.9921, 1.3536) (-24.9921, 4.8197) (-22.2658, 6.7775) (-17.4217, 6.7775) knots 0 0 0 0 1 1 1 1
  spline S668 degree 3 poles (-17.4217, 6.7775) (-14.9356, 6.7775) (-14.1155, 6.2749) (-13.1896, 6.2749) knots 0 0 0 0 1 1 1 1
  spline S669 degree 3 poles (-13.1896, 6.2749) (-12.5264, 6.2749) (-12.315, 6.5129) (-11.8921, 6.5129) knots 0 0 0 0 1 1 1 1
  spline S670 degree 3 poles (-11.8921, 6.5129) (-11.5493, 6.5129) (-11.3378, 6.1954) (-11.2033, 5.6928) knots 0 0 0 0 1 1 1 1
  spline S671 degree 3 poles (-11.2033, 5.6928) (-11.0976, 5.2958) (-10.2518, 1.4065) (-10.2518, 1.195) knots 0 0 0 0 1 1 1 1
  spline S672 degree 3 poles (-10.2518, 1.195) (-10.2518, 0.9833) (-10.8349, 0.4277) (-11.152, 0.4277) knots 0 0 0 0 1 1 1 1
  spline S673 degree 3 poles (-11.152, 0.4277) (-11.655, 0.4277) (-13.8784, 4.8726) (-17.7132, 4.8726) knots 0 0 0 0 1 1 1 1
  line L166 (-130.0537, -8.9121) -> (-127.1702, -4.5202)
  line L167 (-127.1702, -4.5202) -> (-130.0537, -8.9121)
  spline S674 degree 3 poles (167.5457, 6.5131) (167.7547, 6.5131) (168.0193, 5.9575) (168.0193, 5.64) knots 0 0 0 0 1 1 1 1
  spline S675 degree 3 poles (168.0193, 5.64) (168.0193, 5.9575) (167.7547, 6.5131) (167.5457, 6.5131) knots -1 -1 -1 -1 0 0 0 0
  line L168 (2.7113, -9.4149) -> (1.3605, -9.4149)
  line L169 (1.3605, -9.4149) -> (2.7113, -9.4149)
  spline S676 degree 3 poles (218.3166, 6.4337) (219.613, 6.4337) (220.883, 6.4602) (221.9414, 6.5131) knots 0 0 0 0 1 1 1 1
  spline S677 degree 3 poles (221.9414, 6.5131) (220.883, 6.4602) (219.613, 6.4337) (218.3166, 6.4337) knots -1 -1 -1 -1 0 0 0 0
  spline S678 degree 3 poles (-17.5018, -11.5581) (-19.8821, -11.5581) (-20.8625, -11.0288) (-21.7884, -11.0288) knots 0 0 0 0 1 1 1 1
  spline S679 degree 3 poles (-21.7884, -11.0288) (-20.8625, -11.0288) (-19.8821, -11.5581) (-17.5018, -11.5581) knots -1 -1 -1 -1 0 0 0 0
  spline S680 degree 3 poles (311.4213, 5.587) (311.4213, 5.9045) (311.7123, 6.5131) (311.924, 6.4866) knots 0 0 0 0 1 1 1 1
  spline S681 degree 3 poles (311.924, 6.4866) (311.7123, 6.5131) (311.4213, 5.9045) (311.4213, 5.587) knots -1 -1 -1 -1 0 0 0 0
  spline S682 degree 3 poles (297.4505, 5.587) (297.4505, 5.9045) (297.7151, 6.4866) (297.9265, 6.4866) knots 0 0 0 0 1 1 1 1
  spline S683 degree 3 poles (297.9265, 6.4866) (297.7151, 6.4866) (297.4505, 5.9045) (297.4505, 5.587) knots -1 -1 -1 -1 0 0 0 0
  spline S684 degree 3 poles (-11.152, 0.4277) (-11.655, 0.4277) (-13.8784, 4.8726) (-17.7132, 4.8726) knots 0 0 0 0 1 1 1 1
  spline S685 degree 3 poles (-17.7132, 4.8726) (-13.8784, 4.8726) (-11.655, 0.4277) (-11.152, 0.4277) knots -1 -1 -1 -1 0 0 0 0
  line L170 (-46.7651, -8.9652) -> (-46.7651, -0.6308)
  line L171 (-46.7651, -0.6308) -> (-46.7651, -8.9652)
  spline S686 degree 3 poles (-59.2547, -8.9652) (-59.2547, -10.0765) (-57.7986, -9.9971) (-57.7986, -10.4202) knots 0 0 0 0 1 1 1 1
  spline S687 degree 3 poles (-57.7986, -10.4202) (-57.7986, -9.9971) (-59.2547, -10.0765) (-59.2547, -8.9652) knots -1 -1 -1 -1 0 0 0 0
  spline S688 degree 3 poles (189.0272, -10.4203) (189.0272, -10.7378) (188.7626, -11.3225) (188.5245, -11.2934) knots 0 0 0 0 1 1 1 1
  spline S689 degree 3 poles (188.5245, -11.2934) (188.7626, -11.3225) (189.0272, -10.7378) (189.0272, -10.4203) knots -1 -1 -1 -1 0 0 0 0
  spline S690 degree 3 poles (-124.2866, -8.9652) (-123.651, -9.9175) (-125.4494, -10.0233) (-125.4494, -10.4202) knots -1 -1 -1 -1 0 0 0 0
  spline S691 degree 3 poles (-125.4494, -10.4202) (-125.4494, -10.7376) (-125.1587, -11.3224) (-124.9494, -11.2934) knots -1 -1 -1 -1 0 0 0 0
  spline S692 degree 3 poles (-124.9494, -11.2934) (-123.9184, -11.2403) (-122.3565, -11.2139) (-120.8217, -11.2139) knots -1 -1 -1 -1 0 0 0 0
  spline S693 degree 3 poles (-120.8217, -11.2139) (-119.2598, -11.2139) (-117.725, -11.2403) (-116.6669, -11.2934) knots -1 -1 -1 -1 0 0 0 0
  spline S694 degree 3 poles (-116.6669, -11.2934) (-116.4538, -11.3224) (-116.1631, -10.7376) (-116.1631, -10.4202) knots -1 -1 -1 -1 0 0 0 0
  spline S695 degree 3 poles (-116.1631, -10.4202) (-116.1631, -9.9969) (-117.2483, -9.9175) (-117.8839, -8.9652) knots -1 -1 -1 -1 0 0 0 0
  line L172 (-117.8839, -8.9652) -> (-121.8798, -2.8001)
  line L173 (-121.8798, -2.8001) -> (-117.1979, 4.132)
  spline S696 degree 3 poles (-117.1979, 4.132) (-116.5623, 5.0843) (-115.636, 5.2164) (-115.636, 5.6133) knots -1 -1 -1 -1 0 0 0 0
  spline S697 degree 3 poles (-115.636, 5.6133) (-115.636, 5.9311) (-115.9267, 6.5396) (-116.136, 6.5132) knots -1 -1 -1 -1 0 0 0 0
  spline S698 degree 3 poles (-116.136, 6.5132) (-116.5352, 6.4601) (-117.2755, 6.4338) (-118.0157, 6.4338) knots -1 -1 -1 -1 0 0 0 0
  spline S699 degree 3 poles (-118.0157, 6.4338) (-118.756, 6.4338) (-119.4963, 6.4601) (-119.8955, 6.5132) knots -1 -1 -1 -1 0 0 0 0
  spline S700 degree 3 poles (-119.8955, 6.5132) (-120.1048, 6.5396) (-120.4768, 5.9311) (-120.4768, 5.6133) knots -1 -1 -1 -1 0 0 0 0
  spline S701 degree 3 poles (-120.4768, 5.6133) (-120.4768, 5.2164) (-118.9691, 5.0843) (-119.6048, 4.132) knots -1 -1 -1 -1 0 0 0 0
  line L174 (-119.6048, 4.132) -> (-122.9922, -1.0805)
  line L175 (-122.9922, -1.0805) -> (-126.4299, 4.1584)
  spline S702 degree 3 poles (-126.4299, 4.1584) (-127.0384, 5.1106) (-125.2401, 5.2164) (-125.2401, 5.64) knots -1 -1 -1 -1 0 0 0 0
  spline S703 degree 3 poles (-125.2401, 5.64) (-125.2401, 5.9575) (-125.5308, 6.5132) (-125.7439, 6.5132) knots -1 -1 -1 -1 0 0 0 0
  spline S704 degree 3 poles (-125.7439, 6.5132) (-126.802, 6.4601) (-128.3368, 6.4338) (-129.8948, 6.4338) knots -1 -1 -1 -1 0 0 0 0
  spline S705 degree 3 poles (-129.8948, 6.4338) (-131.4296, 6.4338) (-132.9915, 6.4601) (-134.0225, 6.5132) knots -1 -1 -1 -1 0 0 0 0
  spline S706 degree 3 poles (-134.0225, 6.5132) (-134.2356, 6.5132) (-134.5263, 5.9575) (-134.5263, 5.64) knots -1 -1 -1 -1 0 0 0 0
  spline S707 degree 3 poles (-134.5263, 5.64) (-134.5263, 5.2164) (-133.4411, 5.1106) (-132.8326, 4.1584) knots -1 -1 -1 -1 0 0 0 0
  line L176 (-132.8326, 4.1584) -> (-128.3096, -2.7738)
  line L177 (-128.3096, -2.7738) -> (-132.4373, -8.9121)
  spline S708 degree 3 poles (-132.4373, -8.9121) (-133.0729, -9.8648) (-133.9953, -9.9969) (-133.9953, -10.4202) knots -1 -1 -1 -1 0 0 0 0
  spline S709 degree 3 poles (-133.9953, -10.4202) (-133.9953, -10.7376) (-133.7046, -11.3224) (-133.4953, -11.2934) knots -1 -1 -1 -1 0 0 0 0
  spline S710 degree 3 poles (-133.4953, -11.2934) (-133.0961, -11.2403) (-132.3559, -11.2139) (-131.6156, -11.2139) knots -1 -1 -1 -1 0 0 0 0
  spline S711 degree 3 poles (-131.6156, -11.2139) (-130.8754, -11.2139) (-130.1351, -11.2403) (-129.7359, -11.2934) knots -1 -1 -1 -1 0 0 0 0
  spline S712 degree 3 poles (-129.7359, -11.2934) (-129.5266, -11.3224) (-129.1545, -10.7376) (-129.1545, -10.4202) knots -1 -1 -1 -1 0 0 0 0
  spline S713 degree 3 poles (-129.1545, -10.4202) (-129.1545, -9.9969) (-130.6622, -9.8648) (-130.0537, -8.9121) knots -1 -1 -1 -1 0 0 0 0
  line L178 (-130.0537, -8.9121) -> (-127.1702, -4.5202)
  line L179 (-127.1702, -4.5202) -> (-124.2866, -8.9652)
  line L180 (175.9039, -8.965) -> (175.9039, -3.885)
  line L181 (175.9039, -3.885) -> (175.9039, -8.965)
  spline S714 degree 3 poles (-117.8839, -8.9652) (-117.2483, -9.9175) (-116.1631, -9.9969) (-116.1631, -10.4202) knots 0 0 0 0 1 1 1 1
  spline S715 degree 3 poles (-116.1631, -10.4202) (-116.1631, -9.9969) (-117.2483, -9.9175) (-117.8839, -8.9652) knots -1 -1 -1 -1 0 0 0 0
  spline S716 degree 3 poles (188.5245, -11.2934) (187.4661, -11.2405) (186.1961, -11.214) (184.8997, -11.214) knots 0 0 0 0 1 1 1 1
  spline S717 degree 3 poles (184.8997, -11.214) (186.1961, -11.214) (187.4661, -11.2405) (188.5245, -11.2934) knots -1 -1 -1 -1 0 0 0 0
  spline S718 degree 3 poles (180.7986, -10.4203) (180.7986, -10.0234) (182.2539, -10.1028) (182.2539, -8.965) knots 0 0 0 0 1 1 1 1
  spline S719 degree 3 poles (182.2539, -8.965) (182.2539, -10.1028) (180.7986, -10.0234) (180.7986, -10.4203) knots -1 -1 -1 -1 0 0 0 0
  spline S720 degree 3 poles (-120.8217, -11.2139) (-122.3565, -11.2139) (-123.9184, -11.2403) (-124.9494, -11.2934) knots 0 0 0 0 1 1 1 1
  spline S721 degree 3 poles (-124.9494, -11.2934) (-123.9184, -11.2403) (-122.3565, -11.2139) (-120.8217, -11.2139) knots -1 -1 -1 -1 0 0 0 0
  spline S722 degree 3 poles (-43.1421, -5.7371) (-42.6404, -5.7371) (-42.4277, -9.3619) (-38.6427, -9.3619) knots 0 0 0 0 1 1 1 1
  spline S723 degree 3 poles (-38.6427, -9.3619) (-42.4277, -9.3619) (-42.6404, -5.7371) (-43.1421, -5.7371) knots -1 -1 -1 -1 0 0 0 0
  line L182 (-127.1702, -4.5202) -> (-124.2866, -8.9652)
  line L183 (-124.2866, -8.9652) -> (-127.1702, -4.5202)
  spline S724 degree 3 poles (182.2539, -8.965) (182.2539, -10.1028) (180.7986, -10.0234) (180.7986, -10.4203) knots -1 -1 -1 -1 0 0 0 0
  spline S725 degree 3 poles (180.7986, -10.4203) (180.7986, -10.7378) (181.0897, -11.3225) (181.3014, -11.2934) knots -1 -1 -1 -1 0 0 0 0
  spline S726 degree 3 poles (181.3014, -11.2934) (182.3332, -11.2405) (183.6297, -11.214) (184.8997, -11.214) knots -1 -1 -1 -1 0 0 0 0
  spline S727 degree 3 poles (184.8997, -11.214) (186.1961, -11.214) (187.4661, -11.2405) (188.5245, -11.2934) knots -1 -1 -1 -1 0 0 0 0
  spline S728 degree 3 poles (188.5245, -11.2934) (188.7626, -11.3225) (189.0272, -10.7378) (189.0272, -10.4203) knots -1 -1 -1 -1 0 0 0 0
  spline S729 degree 3 poles (189.0272, -10.4203) (189.0272, -9.9969) (187.5984, -10.0763) (187.5984, -8.965) knots -1 -1 -1 -1 0 0 0 0
  line L184 (187.5984, -8.965) -> (187.5984, 4.1583)
  spline S730 degree 3 poles (187.5984, 4.1583) (187.5984, 5.296) (189.0272, 5.2166) (189.0272, 5.64) knots -1 -1 -1 -1 0 0 0 0
  spline S731 degree 3 poles (189.0272, 5.64) (189.0272, 5.9575) (188.7626, 6.5131) (188.5245, 6.5131) knots -1 -1 -1 -1 0 0 0 0
  spline S732 degree 3 poles (188.5245, 6.5131) (187.4661, 6.4602) (186.1961, 6.4337) (184.8997, 6.4337) knots -1 -1 -1 -1 0 0 0 0
  spline S733 degree 3 poles (184.8997, 6.4337) (183.6297, 6.4337) (182.3332, 6.4602) (181.3014, 6.5131) knots -1 -1 -1 -1 0 0 0 0
  spline S734 degree 3 poles (181.3014, 6.5131) (181.0897, 6.5131) (180.7986, 5.9575) (180.7986, 5.64) knots -1 -1 -1 -1 0 0 0 0
  spline S735 degree 3 poles (180.7986, 5.64) (180.7986, 5.2166) (182.2539, 5.296) (182.2539, 4.1583) knots -1 -1 -1 -1 0 0 0 0
  line L185 (182.2539, 4.1583) -> (182.2539, -1.9007)
  line L186 (182.2539, -1.9007) -> (175.9039, -1.9007)
  line L187 (175.9039, -1.9007) -> (175.9039, 4.1583)
  spline S736 degree 3 poles (175.9039, 4.1583) (175.9039, 5.296) (177.3326, 5.2166) (177.3326, 5.64) knots -1 -1 -1 -1 0 0 0 0
  spline S737 degree 3 poles (177.3326, 5.64) (177.3326, 5.9575) (177.068, 6.5131) (176.8564, 6.5131) knots -1 -1 -1 -1 0 0 0 0
  spline S738 degree 3 poles (176.8564, 6.5131) (175.798, 6.4602) (174.5016, 6.4337) (173.2316, 6.4337) knots -1 -1 -1 -1 0 0 0 0
  spline S739 degree 3 poles (173.2316, 6.4337) (171.9351, 6.4337) (170.6386, 6.4602) (169.6068, 6.5131) knots -1 -1 -1 -1 0 0 0 0
  spline S740 degree 3 poles (169.6068, 6.5131) (169.3951, 6.5131) (169.1041, 5.9575) (169.1041, 5.64) knots -1 -1 -1 -1 0 0 0 0
  spline S741 degree 3 poles (169.1041, 5.64) (169.1041, 5.2166) (170.5593, 5.296) (170.5593, 4.1583) knots -1 -1 -1 -1 0 0 0 0
  line L188 (170.5593, 4.1583) -> (170.5593, -8.965)
  spline S742 degree 3 poles (170.5593, -8.965) (170.5593, -10.0763) (169.1041, -9.9969) (169.1041, -10.4203) knots -1 -1 -1 -1 0 0 0 0
  spline S743 degree 3 poles (169.1041, -10.4203) (169.1041, -10.7378) (169.3951, -11.3225) (169.6068, -11.2934) knots -1 -1 -1 -1 0 0 0 0
  spline S744 degree 3 poles (169.6068, -11.2934) (170.6386, -11.2405) (171.9351, -11.214) (173.2316, -11.214) knots -1 -1 -1 -1 0 0 0 0
  spline S745 degree 3 poles (173.2316, -11.214) (174.5016, -11.214) (175.798, -11.2405) (176.8564, -11.2934) knots -1 -1 -1 -1 0 0 0 0
  spline S746 degree 3 poles (176.8564, -11.2934) (177.068, -11.3225) (177.3326, -10.7378) (177.3326, -10.4203) knots -1 -1 -1 -1 0 0 0 0
  spline S747 degree 3 poles (177.3326, -10.4203) (177.3326, -9.9969) (175.9039, -10.0763) (175.9039, -8.965) knots -1 -1 -1 -1 0 0 0 0
  line L189 (175.9039, -8.965) -> (175.9039, -3.885)
  line L190 (175.9039, -3.885) -> (182.2539, -3.885)
  line L191 (182.2539, -3.885) -> (182.2539, -8.965)
  spline S748 degree 3 poles (187.5984, -8.965) (187.5984, -10.0763) (189.0272, -9.9969) (189.0272, -10.4203) knots 0 0 0 0 1 1 1 1
  spline S749 degree 3 poles (189.0272, -10.4203) (189.0272, -9.9969) (187.5984, -10.0763) (187.5984, -8.965) knots -1 -1 -1 -1 0 0 0 0
  spline S750 degree 3 poles (316.3957, 5.587) (316.3957, 5.1902) (315.2051, 5.1902) (314.8347, 4.1318) knots 0 0 0 0 1 1 1 1
  spline S751 degree 3 poles (314.8347, 4.1318) (315.2051, 5.1902) (316.3957, 5.1902) (316.3957, 5.587) knots -1 -1 -1 -1 0 0 0 0
  line L192 (-53.9628, 6.7775) -> (-53.9628, 6.7775)
  line L193 (-53.9628, 6.7775) -> (-53.9628, 6.7775)
  spline S752 degree 3 poles (1.3605, -9.4149) (-1.285, -9.4149) (-2.6606, -8.0125) (-2.6606, -5.949) knots -1 -1 -1 -1 0 0 0 0
  spline S753 degree 3 poles (1.3605, -9.4149) (-1.285, -9.4149) (-2.6606, -8.0125) (-2.6606, -5.949) knots -1 -1 -1 -1 0 0 0 0
  line L194 (-75.2585, 6.5133) -> (-80.6801, -8.9383)
  line L195 (-80.6801, -8.9383) -> (-75.2585, 6.5133)
  spline S754 degree 3 poles (-10.2518, 1.195) (-10.2518, 0.9833) (-10.8349, 0.4277) (-11.152, 0.4277) knots 0 0 0 0 1 1 1 1
  spline S755 degree 3 poles (-11.152, 0.4277) (-10.8349, 0.4277) (-10.2518, 0.9833) (-10.2518, 1.195) knots -1 -1 -1 -1 0 0 0 0
  spline S756 degree 5 poles (-71.5256, -11.2666) (-71.5465, -11.2598) (-71.567, -11.2529) (-71.5869, -11.2458) (-71.6062, -11.2385) (-71.625, -11.231) knots 0 0 0 0 0 0 0.041035 0.041035 0.041035 0.041035 0.041035 0.041035
  spline S757 degree 5 poles (-71.625, -11.231) (-71.6062, -11.2385) (-71.5869, -11.2458) (-71.567, -11.2529) (-71.5465, -11.2598) (-71.5256, -11.2666) knots -0.041035 -0.041035 -0.041035 -0.041035 -0.041035 -0.041035 0 0 0 0 0 0
  spline S758 degree 3 poles (13.3205, 6.1955) (12.7113, 6.1955) (11.3616, 6.6189) (11.3616, 8.4444) knots 0 0 0 0 1 1 1 1
  spline S759 degree 3 poles (11.3616, 8.4444) (11.3616, 6.6189) (12.7113, 6.1955) (13.3205, 6.1955) knots -1 -1 -1 -1 0 0 0 0
  spline S760 degree 3 poles (180.7986, 5.64) (180.7986, 5.9575) (181.0897, 6.5131) (181.3014, 6.5131) knots 0 0 0 0 1 1 1 1
  spline S761 degree 3 poles (181.3014, 6.5131) (181.0897, 6.5131) (180.7986, 5.9575) (180.7986, 5.64) knots -1 -1 -1 -1 0 0 0 0
  line L196 (170.5593, 4.1583) -> (170.5593, -8.965)
  line L197 (170.5593, -8.965) -> (170.5593, 4.1583)
  spline S762 degree 3 poles (-116.136, 6.5132) (-115.9267, 6.5396) (-115.636, 5.9311) (-115.636, 5.6133) knots 0 0 0 0 1 1 1 1
  spline S763 degree 3 poles (-115.636, 5.6133) (-115.636, 5.9311) (-115.9267, 6.5396) (-116.136, 6.5132) knots -1 -1 -1 -1 0 0 0 0
  spline S764 degree 3 poles (169.6068, -11.2934) (169.3951, -11.3225) (169.1041, -10.7378) (169.1041, -10.4203) knots 0 0 0 0 1 1 1 1
  spline S765 degree 3 poles (169.1041, -10.4203) (169.1041, -10.7378) (169.3951, -11.3225) (169.6068, -11.2934) knots -1 -1 -1 -1 0 0 0 0
  spline S766 degree 3 poles (181.3014, 6.5131) (182.3332, 6.4602) (183.6297, 6.4337) (184.8997, 6.4337) knots 0 0 0 0 1 1 1 1
  spline S767 degree 3 poles (184.8997, 6.4337) (183.6297, 6.4337) (182.3332, 6.4602) (181.3014, 6.5131) knots -1 -1 -1 -1 0 0 0 0
  spline S768 degree 3 poles (-129.1545, -10.4202) (-129.1545, -10.7376) (-129.5266, -11.3224) (-129.7359, -11.2934) knots 0 0 0 0 1 1 1 1
  spline S769 degree 3 poles (-129.7359, -11.2934) (-129.5266, -11.3224) (-129.1545, -10.7376) (-129.1545, -10.4202) knots -1 -1 -1 -1 0 0 0 0
  spline S770 degree 3 poles (173.2316, -11.214) (171.9351, -11.214) (170.6386, -11.2405) (169.6068, -11.2934) knots 0 0 0 0 1 1 1 1
  spline S771 degree 3 poles (169.6068, -11.2934) (170.6386, -11.2405) (171.9351, -11.214) (173.2316, -11.214) knots -1 -1 -1 -1 0 0 0 0
  spline S772 degree 3 poles (184.8997, 6.4337) (186.1961, 6.4337) (187.4661, 6.4602) (188.5245, 6.5131) knots 0 0 0 0 1 1 1 1
  spline S773 degree 3 poles (188.5245, 6.5131) (187.4661, 6.4602) (186.1961, 6.4337) (184.8997, 6.4337) knots -1 -1 -1 -1 0 0 0 0
  spline S774 degree 3 poles (-26.6033, -5.7372) (-26.2843, -5.7372) (-25.7028, -6.0017) (-25.7028, -6.2399) knots 0 0 0 0 1 1 1 1
  spline S775 degree 3 poles (-25.7028, -6.2399) (-25.7028, -6.0017) (-26.2843, -5.7372) (-26.6033, -5.7372) knots -1 -1 -1 -1 0 0 0 0
  spline S776 degree 3 poles (214.2155, 5.6135) (214.2155, 5.9575) (214.5066, 6.5131) (214.7182, 6.5131) knots 0 0 0 0 1 1 1 1
  spline S777 degree 3 poles (214.7182, 6.5131) (214.5066, 6.5131) (214.2155, 5.9575) (214.2155, 5.6135) knots -1 -1 -1 -1 0 0 0 0
  spline S778 degree 3 poles (16.2828, -2.3771) (16.2828, 2.518) (17.3668, 4.9254) (19.7498, 4.9254) knots -1 -1 -1 -1 0 0 0 0
  spline S779 degree 3 poles (19.7498, -9.7058) (17.3937, -9.7058) (16.2828, -7.3512) (16.2828, -2.3771) knots -1 -1 -1 -1 0 0 0 0
  spline S780 degree 3 poles (23.2168, -2.3771) (23.2168, -7.2718) (22.1298, -9.7058) (19.7498, -9.7058) knots -1 -1 -1 -1 0 0 0 0
  spline S781 degree 3 poles (19.7498, 4.9254) (22.1298, 4.9254) (23.2168, 2.518) (23.2168, -2.3771) knots -1 -1 -1 -1 0 0 0 0
  ellipse E20 centre (19.5885, -1.7408) end of major axis (19.5885, -11.5568) minor radius 8.5372 (12.3354, 3.4367) -> (19.0342, -11.5361) ccw
  spline S782 degree 3 poles (12.3354, 3.4367) (13.6571, 5.1309) (15.615, 6.2706) (18.0029, 6.6455) knots 0.475314 0.475314 0.475314 0.475314 1 1 1 1
  spline S783 degree 3 poles (18.0029, 6.6455) (17.2638, 6.85) (16.5713, 7.0359) (15.9755, 7.1529) knots 0 0 0 0 0.594925 0.594925 0.594925 0.594925
  spline S784 degree 3 poles (15.9755, 7.1529) (15.5699, 7.2326) (15.2092, 7.2804) (14.9092, 7.2804) knots 0.594925 0.594925 0.594925 0.594925 1 1 1 1
  spline S785 degree 3 poles (14.9092, 7.2804) (13.9565, 7.2804) (13.637, 6.8569) (13.637, 6.2749) knots 0 0 0 0 1 1 1 1
  spline S786 degree 3 poles (13.637, 6.2749) (13.637, 6.2221) (13.5056, 6.1955) (13.3205, 6.1955) knots 0 0 0 0 1 1 1 1
  spline S787 degree 3 poles (13.3205, 6.1955) (12.7113, 6.1955) (11.3616, 6.6189) (11.3616, 8.4444) knots 0 0 0 0 1 1 1 1
  spline S788 degree 3 poles (11.3616, 8.4444) (11.3616, 10.4553) (12.9234, 12.1751) (15.2526, 12.1222) knots 0 0 0 0 1 1 1 1
  spline S789 degree 3 poles (15.2526, 12.1222) (19.1944, 12.0165) (22.2105, 7.307) (24.1426, 7.307) knots 0 0 0 0 1 1 1 1
  spline S790 degree 3 poles (24.1426, 7.307) (24.8832, 7.307) (25.2803, 7.8624) (25.2803, 8.4181) knots 0 0 0 0 1 1 1 1
  spline S791 degree 3 poles (25.2803, 8.4181) (25.2803, 9.0001) (24.9608, 9.5293) (24.0351, 9.5293) knots 0 0 0 0 1 1 1 1